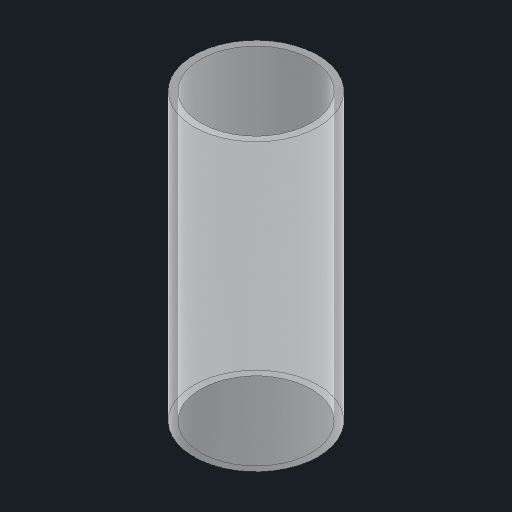
# Autodesk Inventor part: WashChamber
Saved by Autodesk Inventor 2024 (Build 280153000, 153)
## iProperties
Created: 2025-02-06
Part Number: WashChamber
Material: Acrylic, Clear
Document SubType Name: Modeling
Designer: Tommy Rohmann
Density: 1.19 g/cm^3
Appearance: Transparent - Clear
Author: Tommy Rohmann
Autodesk Inventor part; units mm, degrees
ref_plane "YZ Plane" through (0, 0, 0) normal (1, 0, 0) x (0, 1, 0)
ref_plane "XZ Plane" through (0, 0, 0) normal (0, 1, 0) x (-1, 0, 0)
ref_plane "XY Plane" through (0, 0, 0) normal (0, 0, 1) x (1, 0, 0)
sketch "WashChamber" plane through (0, 0, 0) normal (0, 0, 1) x (1, 0, 0)
  line L0 (50.8, 0) -> (50.8, 262.763)
  line L1 (50.8, 262.763) -> (57.15, 262.763)
  line L2 (57.15, 262.763) -> (57.15, 0)
  line L3 (57.15, 0) -> (50.8, 0)
  line L4 (0, 0) -> (0, 172.8328)
  dimension "d2" = 262.763
  dimension "d85" = 114.3
  dimension "d86" = 101.6
  measures "d2" distance of L1.end L2.end
  measures "d85" diameter of L2 L4
  measures "d86" diameter of L0 L4
derived "LAYOUT.ipt"
sketch "Sketch1" plane through (0, 0, 0) normal (0, 0, 1) x (1, 0, 0)
  line L0 (50.8, 0) -> (50.8, 262.763)
  line L1 (50.8, 262.763) -> (57.15, 262.763)
  line L2 (57.15, 262.763) -> (57.15, 0)
  line L3 (57.15, 0) -> (50.8, 0)
  line L4 (0, 0) -> (0, 172.8328)
revolve "Revolution1" add sketch "Sketch1" angle 360 about axis through (0, 0, 0) along (0, 1, 0)
body "Solid1"
